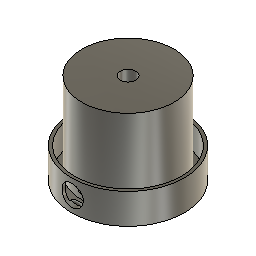
steppermotor v2 (Autodesk Fusion 360 design; units mm, degrees)
Autodesk Fusion 360 part; units mm, degrees
sketch "Sketch6" plane through (0, 0, 0) normal (0, 0, 1) x (1, 0, 0)
  circle A0 centre (0, 0) radius 2.6
  circle A1 centre (0, 0) radius 15.25
  dimension "d35" = 5.2
  dimension "d36" = 30.5
  constraint coincident A0.centre A1.centre
  measures "d35" diameter of A0
  measures "d36" diameter of A1
extrude "Extrude7" add sketch "Sketch6" along normal blind 20
sketch "Sketch7" plane through (0, 0, 0) normal (0, 1, 0) x (1, 0, 0)
  circle A0 centre (0, -5) radius 1.55
  dimension "d39" = 3.1
  measures "d39" diameter of A0
extrude "Extrude8" cut sketch "Sketch7" along normal blind -24 and the other way blind -31
extrude "Extrude9" add 1 faces at (10.9669, -0.8868, 20) along direction (0, 0, 1) blind 10
sketch "Sketch8" plane through (0, 0, 0) normal (0, 0, 1) x (1, 0, 0)
  circle A0 centre (0, 0) radius 2.55
  circle A1 centre (0, 0) radius 18.65
  dimension "d46" = 5.1
  dimension "d47" = 37.3
  constraint coincident A0.centre A1.centre
  measures "d46" diameter of A0
  measures "d47" diameter of A1
extrude "Extrude10" add sketch "Sketch8" along normal blind 2
sketch "Sketch9" plane through (0, 0, 2) normal (0, 0, 1) x (-1, 0, 0)
  circle A0 centre (0, 0) radius 18.65
  circle A1 centre (0, 0) radius 15.25
  circle A2 centre (0, 0) radius 17.65
  dimension "d50" = 35.3
  constraint coincident A0.centre A1.centre
  measures "d50" diameter of A2
extrude "Extrude11" add sketch "Sketch9" along normal blind 25 contours A0
sketch "Sketch10" plane through (0, 0, 0) normal (0, 1, 0) x (1, 0, 0)
  circle A0 through (3.5, -5, -20) (-1.75, -1.9689, -20) (-1.75, -8.0311, -20)
  dimension "d53" = 7
extrude "Extrude12" cut sketch "Sketch10" along normal blind 3 contours A0 in plane through (0, -20, 0) normal (0, 1, 0)
hole "Hole1" at (0, 18.65, 4.8356) direction (0, -1, 0) diameter 7 depth 2 tip angle 180
fillet "Fillet4" radius 1 1 edges at (0, 16.65, 2)
fillet "Fillet5" radius 1 1 edges at (0, -17, 2)
sketch "Sketch11" plane through (0, 0, 30) normal (0, 0, 1) x (-1, 0, 0)
  circle A0 centre (0, 0) radius 2.6
  circle A1 centre (0, 0) radius 15.25
  circle A2 centre (0, 0) radius 17.2919
  circle A3 centre (0, 0) radius 19.8274
  constraint coincident A0.centre A1.centre
  constraint concentric A2 A3
extrude "Extrude13" cut sketch "Sketch11" against normal blind 20 contours A3
